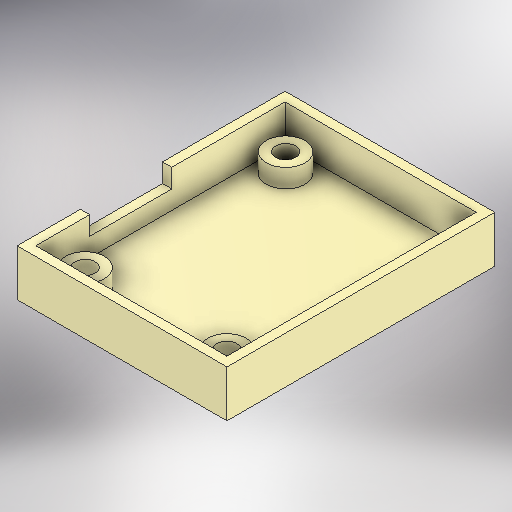
# Autodesk Inventor part: microphone_MCU_case
Saved by Autodesk Inventor 2026 (Build 300175050, 175E)
## iProperties
Created: 2025-06-24
Part Number: microphone_MCU_case
Material: Generic
Document SubType Name: Modeling
Designer: satom
Density: 1 g/cm^3
Appearance: Default
Author: satom
Autodesk Inventor part; units mm, degrees
ref_plane "YZ Plane" through (0, 0, 0) normal (1, 0, 0) x (0, 1, 0)
ref_plane "XZ Plane" through (0, 0, 0) normal (0, 1, 0) x (-1, 0, 0)
ref_plane "XY Plane" through (0, 0, 0) normal (0, 0, 1) x (1, 0, 0)
sketch "Sketch1" plane through (0, 0, 0) normal (0, 1, 0) x (-1, 0, 0)
  line L0 (16.3, 21.25) -> (-16.3, 21.25)
  line L1 (-16.3, 21.25) -> (-16.3, -21.25)
  line L2 (-16.3, -21.25) -> (16.3, -21.25)
  line L3 (16.3, -21.25) -> (16.3, 21.25)
  line L4 (16.3, 21.25) -> (-16.3, -21.25) construction
  line L5 (-16.3, 21.25) -> (16.3, -21.25) construction
  circle A0 centre (12.1, 17.05) radius 1.7
  circle A1 centre (12.1, -17.15) radius 1.7
  circle A2 centre (-12.1, 17.05) radius 1.7
  point P0 (0, 0)
  dimension "d0" = 42.5
  dimension "d1" = 32.6
  dimension "d4" = 3.4
  dimension "d5" = 3.4
  dimension "d6" = 3.4
  dimension "d7" = 34.2
  dimension "d8" = 24.2
  dimension "d9" = 4.2
  dimension "d10" = 4.2
  dimension "d11" = 4.2
  dimension "d12" = 4.2
  constraints: 12 end point, 3 centre point, 2 midpoint, 2 parallel, 1 horizontal, 1 perpendicular
  measures "d0" distance of L0.end L1.end
  measures "d1" distance of L1.end L2.end
  measures "d4" diameter of A0
  measures "d5" diameter of A1
  measures "d6" diameter of A2
  measures "d7" distance of A1.centre A0.centre
  measures "d8" distance of A2.centre A0.centre
  measures "d9" distance from line of L3 A1.centre
  measures "d10" distance from line of L3 A0.centre
  measures "d11" distance from line of L0 A0.centre
  measures "d12" distance from line of L0 A2.centre
extrude "Extrusion1" add sketch "Sketch1" along normal blind 1.5875
sketch "Sketch2" plane through (0, 1.5875, 0) normal (0, 1, 0) x (1, 0, 0)
  circle A0 centre (-12.1, -17.05) radius 1.7 projected
  circle A1 centre (-12.1, -17.05) radius 1.7
  circle A2 centre (-12.1, -17.05) radius 3.2875
  circle A3 centre (12.1, -17.05) radius 1.7 projected
  circle A4 centre (12.1, -17.05) radius 1.7
  circle A5 centre (12.1, -17.05) radius 3.2875
  circle A6 centre (-12.1, 17.15) radius 1.7 projected
  circle A7 centre (-12.1, 17.15) radius 1.7
  circle A8 centre (-12.1, 17.15) radius 3.2875
  point P0 (0, 0)
  dimension "d13" = 1.5875
  dimension "d14" = 1.5875
  dimension "d15" = 1.5875
  constraints: 6 centre point, 6 coincident
  measures "d13" radial gap between concentric circles of A2 A0
  measures "d14" radial gap between concentric circles of A6 A8
  measures "d15" radial gap between concentric circles of A5 A4
extrude "Extrusion2" add sketch "Sketch2" along normal blind 3.175
sketch "Sketch3" plane through (0, 0, 0) normal (0, -1, 0) x (1, 0, 0)
  line L0 (17.8875, 22.8375) -> (-17.8875, 22.8375)
  line L1 (-17.8875, 22.8375) -> (-17.8875, -22.8375)
  line L2 (-17.8875, -22.8375) -> (17.8875, -22.8375)
  line L3 (17.8875, -22.8375) -> (17.8875, 22.8375)
  line L4 (17.8875, 22.8375) -> (-17.8875, -22.8375) construction
  line L5 (-17.8875, 22.8375) -> (17.8875, -22.8375) construction
  line L6 (16.3, -21.25) -> (-16.3, -21.25) projected
  line L7 (16.3, 21.25) -> (16.3, -21.25) projected
  line L8 (-16.3, 21.25) -> (16.3, 21.25)
  line L9 (16.3, 21.25) -> (16.3, -21.25)
  line L10 (16.3, -21.25) -> (-16.3, -21.25)
  line L11 (-16.3, -21.25) -> (-16.3, 21.25)
  line L12 (-16.3, 21.25) -> (16.3, -21.25) construction
  line L13 (16.3, 21.25) -> (-16.3, -21.25) construction
  point P0 (0, 0)
  point P1 (-16.3, -21.25)
  dimension "d18" = 1.5875
  dimension "d19" = 1.5875
  dimension "d26" = 35.775
  dimension "d27" = 45.675
  constraints: 24 end point, 4 midpoint, 4 parallel, 2 horizontal, 2 perpendicular
  measures "d18" distance between parallel lines of L2 L6
  measures "d19" distance between parallel lines of L3 L7
  measures "d26" distance of L0.start L0.end
  measures "d27" distance of L0.end L1.end
extrude "Extrusion3" add sketch "Sketch3" against normal blind 7.9625
sketch "Sketch4" plane through (0, 7.9625, 0) normal (0, 1, 0) x (1, 0, 0)
  line L0 (-16.3, 21.25) -> (-16.3, -21.25) projected
  line L1 (-17.8875, -22.8375) -> (-17.8875, 22.8375) projected
  line L2 (-16.3, -12.05) -> (-17.8875, -12.05)
  line L3 (-17.8875, -12.05) -> (-17.8875, 1.95)
  line L4 (-17.8875, 1.95) -> (-16.3, 1.95)
  line L5 (-16.3, 1.95) -> (-16.3, -12.05)
  circle A0 centre (-12.1, -17.05) radius 1.7 construction
  circle A1 centre (-12.1, -17.05) radius 1.7 construction
  point P0 (0, 0)
  point P1 (-17.0938, -12.05)
  point P2 (-17.0938, 1.95)
  dimension "d22" = 5
  dimension "d23" = 14
  constraints: 8 end point, 2 midpoint, 2 parallel, 2 point on line, 1 centre point, 1 coincident, 1 horizontal, 1 perpendicular
  measures "d22" vertical distance of L2.start A1.centre
  measures "d23" distance of point (-17.094, -12.05) point (-17.094, 1.95)
extrude "Extrusion4" cut sketch "Sketch4" against normal blind 3.2
equation "\"d4\" = m3_clearance"
equation "\"d5\" = m3_clearance"
equation "\"d6\" = m3_clearance"
equation "\"d10\" = d9"
equation "\"d11\" = d9"
equation "\"d12\" = d9"
equation "\"d14\" = d13"
equation "\"d15\" = d13"
equation "\"m3_heat_set_insert\" = 4"
equation "\"m3_clearance\" = 3.4"
equation "\"m3_heat_set_depth\" = 7"
equation "\"robot_diameter\" = 354"
equation "\"hardboard_thickness\" = 5"
equation "\"motor_centerline_height\" = 13"
body "Solid1"
